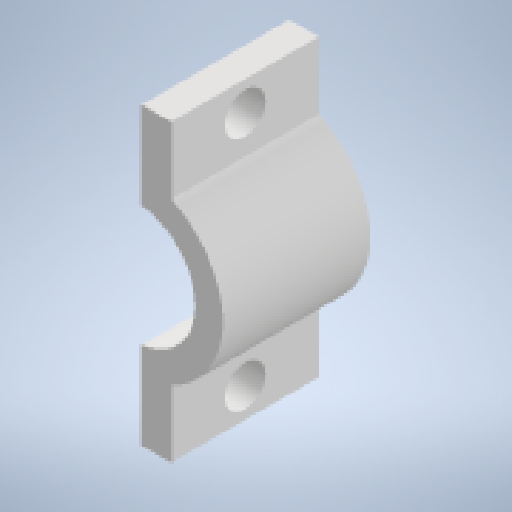
# Autodesk Inventor part: RobotarmHolderSpaende
Saved by Autodesk Inventor 2025.1 (Build 291241000, 241)
## iProperties
Created: 2025-03-06
Part Number: RobotarmHolderSpaende
Material: Generic
Document SubType Name: Modeling
Designer: frede
Density: 1 g/cm^3
Appearance: Default
Author: frede
Autodesk Inventor part; units mm, degrees
ref_plane "YZ Plane" through (0, 0, 0) normal (1, 0, 0) x (0, 1, 0)
ref_plane "XZ Plane" through (0, 0, 0) normal (0, 1, 0) x (-1, 0, 0)
ref_plane "XY Plane" through (0, 0, 0) normal (0, 0, 1) x (1, 0, 0)
sketch "Sketch1" plane through (0, 0, 0) normal (0, 0, 1) x (1, 0, 0)
  line L0 (-1, 20) -> (-1, -20)
  line L1 (-1, -20) -> (1, 20) construction
  line L2 (1, -20) -> (-1, 20) construction
  line L3 (-5, 20) -> (-5, -20)
  line L4 (-5, -20) -> (5, 20) construction
  line L5 (5, -20) -> (-5, 20) construction
  line L6 (-5, -20) -> (-1, -20)
  line L7 (1, -20) -> (5, -20)
  line L8 (5, 20) -> (1, 20)
  line L9 (-1, 20) -> (-5, 20)
  arc A0 (-1, 11.9583) -> (-1, -11.9583) centre (0, 0) ccw
  arc A1 (-1, 8.1892) -> (-1, -8.1892) centre (0, 0) ccw
  arc A2 (1, -8.1892) -> (1, 8.1892) centre (0, 0) ccw
  line L10 (5, -20) -> (5, -10.9087)
  line L11 (5, 10.9087) -> (5, 20)
  line L12 (1, -20) -> (1, -8.1892)
  line L13 (1, 8.1892) -> (1, 20)
  arc A3 (5, -10.9087) -> (5, 10.9087) centre (0, 0) ccw
  dimension "d2" = 2
  dimension "d3" = 40
  dimension "d4" = 10
  constraints: 28 end point, 8 parallel, 8 point on circle, 4 centre point, 4 midpoint, 4 perpendicular, 4 point on line, 2 coincident, 2 horizontal
  measures "d2" distance of L0.start L1.end
  measures "d3" distance of L1.end L2.start
  measures "d4" distance of L3.start L4.end
extrude "Extrusion1" add sketch "Sketch1" along normal blind 20 contours L12 A2 L13 L8 L11 A3 L10 L7
sketch "Sketch2" plane through (1, 8.1892, 0) normal (-1, 0, 0) x (0, 0, 1)
  circle A0 centre (10, 7.8108) radius 2.75
  circle A1 centre (10, -24.1892) radius 2.75
  line L0 (0, -28.1892) -> (20, -28.1892) projected
  line L1 (0, 11.8108) -> (20, 11.8108) projected
  line L2 (20, 11.8108) -> (20, 0) projected
  line L3 (0, 11.8108) -> (0, 0) projected
  line L4 (0, -16.3783) -> (0, -28.1892) projected
  point P0 (0, -8.1892)
  point P1 (0, 5.9054)
  dimension "d9" = 5.5
  dimension "d10" = 5.5
  dimension "d11" = 40
  dimension "d12" = 20
  dimension "d13" = 10
  dimension "d14" = 10
  dimension "d15" = 32
  dimension "d16" = 4
  constraints: 2 centre point, 1 midpoint
  measures "d9" diameter of A0
  measures "d10" diameter of A1
  measures "d11" distance between parallel lines of L0 L1
  measures "d12" distance between parallel lines of L2 L3
  measures "d13" horizontal distance of point (0, 5.905) A0.centre
  measures "d14" distance from line of L4 A1.centre
  measures "d15" distance of A1.centre A0.centre
  measures "d16" distance from line of L1 A0.centre
extrude "Extrusion2" cut sketch "Sketch2" against normal up to surface (4 mm away)
equation "\"d10\" = d9"
equation "\"d16\" = -0.5 * d15 + 0.5 * d11"
body "Solid1"
